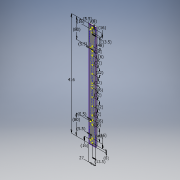
# Autodesk Inventor part: MCbeamdimensions
Saved by Autodesk Inventor 2016 (Build 200138000, 138)
## iProperties
Created: 2015-09-04
Part Number: MCbeamdimensions
Material: Generic
Document SubType Name: Modeling
Designer: Tim
Density: 1 g/cm^3
Appearance: Default
Author: Tim
Autodesk Inventor part; units mm, degrees
ref_plane "YZ Plane" through (0, 0, 0) normal (1, 0, 0) x (0, 1, 0)
ref_plane "XZ Plane" through (0, 0, 0) normal (0, 1, 0) x (-1, 0, 0)
ref_plane "XY Plane" through (0, 0, 0) normal (0, 0, 1) x (1, 0, 0)
sketch "Sketch1" plane through (0, 0, 0) normal (0, 1, 0) x (-1, 0, 0)
  line L0 (-13.5, 208) -> (13.5, 208)
  line L1 (13.5, 208) -> (13.5, -208)
  line L2 (13.5, -208) -> (-13.5, -208)
  line L3 (-13.5, -208) -> (-13.5, 208)
  line L4 (-13.5, 208) -> (13.5, -208) construction
  line L5 (13.5, 208) -> (-13.5, -208) construction
  circle A0 centre (0, 200) radius 1.85 projected
  circle A1 centre (0, 184) radius 1.85 projected
  circle A2 centre (0, 136) radius 1.85 projected
  circle A3 centre (0, 120) radius 1.85 projected
  circle A4 centre (0, 104) radius 1.85 projected
  circle A5 centre (0, 72) radius 1.85 projected
  circle A6 centre (0, 40) radius 1.85 projected
  circle A7 centre (0, 8) radius 1.85 projected
  circle A8 centre (0, 8) radius 1.85 projected
  circle A9 centre (0, -8) radius 1.85 projected
  circle A10 centre (0, -40) radius 1.85 projected
  circle A11 centre (0, -72) radius 1.85 projected
  circle A12 centre (0, -104) radius 1.85 projected
  circle A13 centre (0, -120) radius 1.85 projected
  circle A14 centre (0, -136) radius 1.85 projected
  circle A15 centre (0, -184) radius 1.85 projected
  circle A16 centre (0, -200) radius 1.85 projected
  circle A17 centre (8, -192) radius 1.85 projected
  circle A18 centre (8, -128) radius 1.85 projected
  circle A19 centre (8, 192) radius 1.85 projected
  circle A20 centre (8, 128) radius 1.85 projected
  point P0 (0, 0)
  dimension "d0" = 27
  dimension "d1" = 416
  dimension "d14" = 8
  dimension "d15" = 5.5
  dimension "d16" = 13.5
  dimension "d17" = 16
  dimension "d18" = 80
  dimension "d19" = 16
  dimension "d20" = 80
  dimension "d21" = 16
  dimension "d22" = 5.5
  dimension "d23" = 5.5
  dimension "d24" = 8
  dimension "d25" = 13.5
  dimension "d26" = 16
  dimension "d27" = 16
  dimension "d28" = 16
  dimension "d29" = 32
  dimension "d30" = 32
  dimension "d31" = 32
  dimension "d32" = 16
  dimension "d33" = 32
  dimension "d34" = 32
  dimension "d35" = 32
  dimension "d36" = 16
  dimension "d37" = 16
  dimension "d38" = 48
  dimension "d39" = 48
  dimension "d40" = 5.5
  constraints: 12 end point, 2 midpoint, 2 parallel, 1 horizontal, 1 perpendicular
  measures "d0" distance of L1.end L2.end
  measures "d1" distance of L0.end L1.end
  measures "d14" distance from line of L0 A0.centre
  measures "d15" distance from line of L1 A19.centre
  measures "d16" distance from line of L3 A0.centre
  measures "d17" distance from line of L0 A19.centre
  measures "d18" distance from line of L0 A20.centre
  measures "d19" distance of A1.centre A0.centre
  measures "d20" distance from line of L2 A18.centre
  measures "d21" distance from line of L2 A17.centre
  measures "d22" distance from line of L1 A18.centre
  measures "d23" distance from line of L1 A17.centre
  measures "d24" distance from line of L2 A16.centre
  measures "d25" distance from line of L3 A16.centre
  measures "d26" distance of A16.centre A15.centre
  measures "d27" distance of A13.centre A14.centre
  measures "d28" distance of A12.centre A13.centre
  measures "d29" distance of A12.centre A11.centre
  measures "d30" distance of A11.centre A10.centre
  measures "d31" distance of A10.centre A9.centre
  measures "d32" distance of A9.centre A7.centre
  measures "d33" distance of A7.centre A6.centre
  measures "d34" distance of A5.centre A6.centre
  measures "d35" distance of A4.centre A5.centre
  measures "d36" distance of A3.centre A4.centre
  measures "d37" distance of A3.centre A2.centre
  measures "d38" distance of A15.centre A14.centre
  measures "d39" distance of A2.centre A1.centre
  measures "d40" distance from line of L1 A20.centre
extrude "Extrusion6" add sketch "Sketch1" along normal blind 6
body "Solid5"
